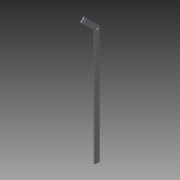
# Autodesk Inventor part: Cart Handle
Saved by Autodesk Inventor 2014 SP1 (Build 180222100, 222)
## iProperties
Created: 2014-02-04
Part Number: Cart Handle
Material: Generic
Document SubType Name: Modeling
Designer: Nitesh
Density: 1 g/cm^3
Appearance: Default
Mass: 115.401 g
Surface Area: 462.152 cm^2
Volume: 115.401 cm^3
Author: Nitesh
Autodesk Inventor part; units mm, degrees
ref_plane "YZ Plane" through (0, 0, 0) normal (1, 0, 0) x (0, 1, 0)
ref_plane "XZ Plane" through (0, 0, 0) normal (0, 1, 0) x (-1, 0, 0)
ref_plane "XY Plane" through (0, 0, 0) normal (0, 0, 1) x (1, 0, 0)
sketch "Sketch1" plane through (0, 0, 0) normal (1, 0, 0) x (0, 1, 0)
  line L0 (0, 25.4) -> (0, 0)
  line L1 (0, 25.4) -> (609.6, 25.4)
  line L2 (609.6, 25.4) -> (681.442, 97.242)
  line L3 (681.442, 97.242) -> (632.8429, 48.6429)
  line L4 (681.442, 97.242) -> (699.4026, 79.2815)
  line L5 (699.4026, 79.2815) -> (620.121, 0)
  line L6 (0, 0) -> (620.121, 0)
  line L7 (609.6, 25.4) -> (620.121, 0) construction
  circle A0 centre (614.8605, 12.7) radius 6.35
  circle A1 centre (681.442, 79.2815) radius 3.175
  dimension "d0" = 25.4
  dimension "d7" = 609.6
  dimension "d8" = 101.6
  dimension "d9" = 135
  dimension "d10" = 25.4
  dimension "d11" = 12.7
  dimension "d12" = 6.35
  dimension "d13" = 12.7
  dimension "d14" = 12.7
  constraints: 16 end point, 3 perpendicular, 2 centre point, 1 midpoint, 1 parallel, 1 point on line, 1 vertical
  measures "d0" distance of L0.start L0.end
  measures "d7" distance of L0.start L1.end
  measures "d8" distance of L1.end L2.end
  measures "d9" angle of L1 L2
  measures "d10" distance of L2.end L4.end
  measures "d11" diameter of A0
  measures "d12" diameter of A1
  measures "d13" distance from line of L4 A1.centre
  measures "d14" distance from line of L5 A1.centre
extrude "Extrusion1" add sketch "Sketch1" along normal blind 6.35
body "Solid1"
